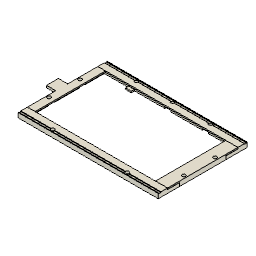
toshiba-screen-frame (Autodesk Fusion 360 design; units mm, degrees)
part number: 2026-06-13-12-57-34-662
part number: 2026-06-16-20-14-57-476
part number: 2026-06-16-20-14-57-486
part number: 2026-06-16-20-14-57-489
part number: 2026-06-16-20-14-57-492
part number: 2026-06-18-16-57-17-201
Autodesk Fusion 360 part; units mm, degrees
note: some values were not read from the file. Chosen so that the rebuilt part matches the saved one: which bodies a step acts on; which face or edge a step refers to. Set by a fixed rule: which sketch regions a step uses.
sketch "Main" plane through (0, 0, 0) normal (0, 1, 0) x (1, 0, 0)
  line L0 (0, 0) -> (200, 0)
  line L1 (200, 0) -> (200, -117)
  line L2 (200, -117) -> (0, -117)
  line L3 (0, -117) -> (0, 0)
  line L4 (-5, 3) -> (207, 3)
  line L5 (207, 3) -> (207, -124)
  line L6 (207, -124) -> (-5, -124)
  line L7 (-5, -124) -> (-5, 3)
  line L8 (-13, 15.5) -> (220.2, 15.5)
  line L9 (220.2, 15.5) -> (220.2, -132.5)
  line L10 (220.2, -132.5) -> (-13, -132.5)
  line L11 (-13, -132.5) -> (-13, 15.5)
  dimension "d1" = 200
  dimension "d2" = 117
  dimension "d4" = 127
  dimension "d5" = 3
  dimension "d6" = 5
  dimension "d7" = 148
  dimension "d9" = 12.5
  dimension "d10" = 8
  dimension "d37" = 7
  dimension "d38" = 212
  dimension "d39" = 13.2
  dimension "d40" = 233.2
  constraint horizontal L0
  constraint vertical L1
  constraint horizontal L2
  constraint vertical L3
  constraint coincident L0.start L3.end
  constraint horizontal L4
  constraint vertical L5
  constraint horizontal L6
  constraint vertical L7
  constraint horizontal L8
  constraint vertical L9
  constraint horizontal L10
  constraint vertical L11
  measures "d1" distance of L0.start L0.end
  measures "d2" distance of L0.start L2.end
  measures "d4" distance of L4.start L6.end
  measures "d5" distance of L0 L4
  measures "d6" distance of L3 L7
  measures "d7" distance of L8.start L10.end
  measures "d9" distance of L4 L8
  measures "d10" distance of L7 L11
  measures "d37" distance of L1 L5
  measures "d38" distance of L5 L7
  measures "d39" distance of L5 L9
  measures "d40" distance of L9 L11
extrude "Extrude1" add sketch "Main" against normal blind 7.9 contours L8 L9 L10 L11 makes body 1
extrude "Extrude2" add sketch "Main" against normal blind 2 contours L4 L5 L6 L7 bodies 1
sketch "Notches" plane through (0, -7.9, 0) normal (0, -1, 0) x (1, 0, 0)
  line L0 (-5, 124) -> (207, 124)
  line L1 (207, 124) -> (207, -3)
  line L2 (207, -3) -> (-5, -3)
  line L3 (-5, -3) -> (-5, 124)
  line L4 (220.2, 132.5) -> (-13, 132.5)
  line L5 (-13, 132.5) -> (-13, -15.5)
  line L6 (-13, -15.5) -> (220.2, -15.5)
  line L7 (220.2, -15.5) -> (220.2, 132.5)
  line L8 (35.1303, -3) -> (45.1303, -3)
  line L9 (45.1303, -3) -> (45.1303, -14)
  line L10 (45.1303, -14) -> (35.1303, -14)
  line L11 (35.1303, -14) -> (35.1303, -3)
  line L12 (95.4758, -3) -> (105.4758, -3)
  line L13 (105.4758, -3) -> (105.4758, -14)
  line L14 (105.4758, -14) -> (95.4758, -14)
  line L15 (95.4758, -14) -> (95.4758, -3)
  line L16 (158.4262, -3) -> (168.4262, -3)
  line L17 (168.4262, -3) -> (168.4262, -14)
  line L18 (168.4262, -14) -> (158.4262, -14)
  line L19 (158.4262, -14) -> (158.4262, -3)
  line L20 (-12, 90) -> (-5, 90)
  line L21 (-5, 90) -> (-5, 80)
  line L22 (-5, 80) -> (-12, 80)
  line L23 (-12, 80) -> (-12, 90)
  line L24 (-12, 38.3982) -> (-5, 38.3982)
  line L25 (-5, 38.3982) -> (-5, 28.3982)
  line L26 (-5, 28.3982) -> (-12, 28.3982)
  line L27 (-12, 28.3982) -> (-12, 38.3982)
  line L28 (34.9856, 124) -> (44.9856, 124)
  line L29 (44.9856, 124) -> (44.9856, 131)
  line L30 (44.9856, 131) -> (34.9856, 131)
  line L31 (34.9856, 131) -> (34.9856, 124)
  line L32 (158.8604, 124) -> (168.8604, 124)
  line L33 (168.8604, 124) -> (168.8604, 131)
  line L34 (168.8604, 131) -> (158.8604, 131)
  line L35 (158.8604, 131) -> (158.8604, 124)
  line L36 (207, 90.4116) -> (218.7, 90.4116)
  line L37 (218.7, 90.4116) -> (218.7, 80.4116)
  line L38 (218.7, 80.4116) -> (207, 80.4116)
  line L39 (207, 80.4116) -> (207, 90.4116)
  line L40 (207, 38.4594) -> (218.7, 38.4594)
  line L41 (218.7, 38.4594) -> (218.7, 28.4594)
  line L42 (218.7, 28.4594) -> (207, 28.4594)
  line L43 (207, 28.4594) -> (207, 38.4594)
  dimension "d15" = 10
  dimension "d17" = 10
  dimension "d19" = 10
  dimension "d21" = 10
  dimension "d22" = 10
  dimension "d23" = 10
  dimension "d27" = 10
  dimension "d29" = 10
  dimension "d30" = 10
  dimension "d62" = 1.5
  dimension "d63" = 1.5
  dimension "d64" = 1.5
  dimension "d65" = 1.5
  dimension "d66" = 1.5
  dimension "d67" = 1.5
  dimension "d68" = 1.5
  dimension "d71" = 7
  dimension "d72" = 7
  constraint horizontal L8
  constraint vertical L9
  constraint horizontal L10
  constraint vertical L11
  constraint horizontal L12
  constraint vertical L13
  constraint horizontal L14
  constraint vertical L15
  constraint horizontal L16
  constraint vertical L17
  constraint horizontal L18
  constraint vertical L19
  constraint horizontal L20
  constraint vertical L21
  constraint horizontal L22
  constraint vertical L23
  constraint horizontal L24
  constraint vertical L25
  constraint horizontal L26
  constraint vertical L27
  constraint horizontal L28
  constraint vertical L29
  constraint horizontal L30
  constraint vertical L31
  constraint horizontal L32
  constraint vertical L33
  constraint horizontal L34
  constraint vertical L35
  constraint horizontal L36
  constraint vertical L37
  constraint horizontal L38
  constraint vertical L39
  constraint horizontal L40
  constraint vertical L41
  constraint horizontal L42
  constraint vertical L43
  constraint collinear L2 L16
  constraint collinear L2 L8
  constraint collinear L2 L12
  constraint collinear L1 L43
  constraint collinear L1 L39
  constraint collinear L0 L32
  constraint collinear L0 L28
  constraint collinear L3 L25
  constraint collinear L3 L21
  measures "d15" distance of L8.start L8.end
  measures "d17" distance of L12.start L12.end
  measures "d19" distance of L16.start L16.end
  measures "d21" distance of L20.start L22.end
  measures "d22" distance of L24.start L26.end
  measures "d23" distance of L28.start L28.end
  measures "d27" distance of L32.start L32.end
  measures "d29" distance of L36.start L38.end
  measures "d30" distance of L40.start L42.end
  measures "d62" distance of L6 L18
  measures "d63" distance of L6 L14
  measures "d64" distance of L6 L10
  measures "d65" distance of L7 L41
  measures "d66" distance of L7 L37
  measures "d67" distance of L4 L34
  measures "d68" distance of L4 L30
  measures "d71" distance of L25 L27
  measures "d72" distance of L21 L23
extrude "Extrude3" cut sketch "Notches" against normal blind 2.3 contours L3 L20 L21 L22 L23 bodies 1
extrude "Extrude4" cut sketch "Notches" against normal blind 2.3 contours L0 L28 L29 L30 L31 | L0 L32 L33 L34 L35 | L3 L24 L25 L26 L27 | L1 L36 L37 L38 L39 | L2 L8 L9 L10 L11 | L1 L40 L41 L42 L43 | L2 L12 L13 L14 L15 | L2 L16 L17 L18 L19 bodies 1
ref_plane "WorkPlane1" through (103.6, -3.95, 102.5) normal (0, 0, 1) x (-1, 0, 0)
split "Split1" by plane through (103.6, -3.95, 102.5) normal (0, 0, 1) bodies 1 makes body 2 at (135.7333, 0, 127.3333)
ref_plane "WorkPlane2" through (103.6, -3.95, 14.5) normal (0, 0, -1) x (1, 0, 0)
split "Split2" by plane through (103.6, -3.95, 14.5) normal (0, 0, -1) bodies 1 makes body 3 at (206.7333, 0, 43.8333) makes body 4 at (135.7333, 0, -10.3333)
sketch "channels" plane through (220.2, 0, 0) normal (1, 0, 0) x (0, 0, -1)
  line L0 (-14.5, 0) -> (-14.5, -7.9)
  line L1 (-14.5, -7.9) -> (15.5, -7.9)
  line L2 (15.5, -7.9) -> (15.5, 0)
  line L3 (15.5, 0) -> (-14.5, 0)
  line L4 (14.5, 0) -> (11, 0)
  line L5 (11, 0) -> (11, -1)
  line L6 (11, -1) -> (14.5, -1)
  line L7 (14.5, -1) -> (14.5, 0)
  line L8 (-131.5, 0) -> (-128, 0)
  line L9 (-128, 0) -> (-128, -1)
  line L10 (-128, -1) -> (-131.5, -1)
  line L11 (-131.5, -1) -> (-131.5, 0)
  line L12 (-132.5, 0) -> (-132.5, -7.9)
  dimension "d41" = 3.5
  dimension "d42" = 1
  dimension "d43" = 1
  dimension "d44" = 3.5
  dimension "d45" = 1
  dimension "d46" = 1
  constraint horizontal L4
  constraint vertical L5
  constraint horizontal L6
  constraint vertical L7
  constraint coincident L3 L4.start
  constraint horizontal L8
  constraint vertical L9
  constraint horizontal L10
  constraint vertical L11
  measures "d41" distance of L4.start L4.end
  measures "d42" distance of L4.start L6.end
  measures "d43" distance of L2 L7
  measures "d44" distance of L8.start L8.end
  measures "d45" distance of L8.start L10.end
  measures "d46" distance of L11 L12
extrude "Extrude5" cut sketch "channels" against normal up to surface (233.2 mm away) contours L3 L4 L5 L6 L7 bodies 4
extrude "Extrude6" cut sketch "channels" against normal up to surface (233.2 mm away) contours L8 L9 L10 L11 bodies 2
combine "Combine1" operation add target body 4 tool bodies 3 2 1
ref_plane "WorkPlane5" through (163.4262, -4.1, -8.5) normal (0, -1, 0) x (0, 0, -1)
sketch "Screws Nuts" plane through (0, -4.1, 0) normal (0, -1, 0) x (-1, 0, 0)
  circle A0 centre (-163.4262, 11) radius 1.6
  circle A1 centre (-163.4262, 11) radius 2.85
  line L0 (-168.4262, 14) -> (-158.4262, 14)
  line L1 (-168.4262, 3) -> (-168.4262, 14)
  circle A2 centre (-100.4758, 11) radius 1.6
  circle A3 centre (-100.4758, 11) radius 2.85
  circle A4 centre (-40.1303, 11) radius 1.6
  circle A5 centre (-40.1303, 11) radius 2.85
  circle A6 centre (9, -33.3982) radius 1.6
  circle A7 centre (9, -33.3982) radius 2.85
  circle A8 centre (-215.7, -33.4594) radius 1.6
  circle A9 centre (-215.7, -33.4594) radius 2.85
  circle A10 centre (9, -85) radius 1.6
  circle A11 centre (9, -85) radius 2.85
  circle A12 centre (-215.7, -85.4116) radius 1.6
  circle A13 centre (-215.7, -85.4116) radius 2.85
  circle A14 centre (-163.8604, -128) radius 1.6
  circle A15 centre (-163.8604, -128) radius 2.85
  circle A16 centre (-39.9856, -128) radius 1.6
  circle A17 centre (-39.9856, -128) radius 2.85
  line L2 (-105.4758, 14) -> (-95.4758, 14)
  line L3 (-105.4758, 3) -> (-105.4758, 14)
  line L4 (-45.1303, 14) -> (-35.1303, 14)
  line L5 (-45.1303, 3) -> (-45.1303, 14)
  line L6 (12, -28.3982) -> (12, -38.3982)
  line L7 (5, -28.3982) -> (12, -28.3982)
  line L8 (12, -80) -> (12, -90)
  line L9 (5, -80) -> (12, -80)
  line L10 (-44.9856, -131) -> (-34.9856, -131)
  line L11 (-44.9856, -124) -> (-44.9856, -131)
  line L12 (-168.8604, -131) -> (-158.8604, -131)
  line L13 (-168.8604, -124) -> (-168.8604, -131)
  line L14 (-218.7, -90.4116) -> (-218.7, -80.4116)
  line L15 (-218.7, -80.4116) -> (-207, -80.4116)
  line L16 (-218.7, -38.4594) -> (-218.7, -28.4594)
  line L17 (-218.7, -28.4594) -> (-207, -28.4594)
  dimension "d74" = 3.2
  dimension "d75" = 5.7
  dimension "d76" = 3
  dimension "d77" = 5
  dimension "d82" = 3.2
  dimension "d83" = 5.7
  dimension "d84" = 3.2
  dimension "d85" = 5.7
  dimension "d86" = 3.2
  dimension "d87" = 5.7
  dimension "d88" = 3.2
  dimension "d89" = 5.7
  dimension "d90" = 3.2
  dimension "d91" = 5.7
  dimension "d92" = 3.2
  dimension "d93" = 5.7
  dimension "d94" = 3.2
  dimension "d95" = 5.7
  dimension "d96" = 3.2
  dimension "d97" = 5.7
  dimension "d98" = 3
  dimension "d99" = 5
  dimension "d100" = 3
  dimension "d101" = 5
  dimension "d102" = 3
  dimension "d103" = 5
  dimension "d104" = 3
  dimension "d105" = 5
  dimension "d106" = 3
  dimension "d107" = 5
  dimension "d108" = 3
  dimension "d109" = 5
  dimension "d110" = 3
  dimension "d111" = 5
  dimension "d112" = 3
  dimension "d113" = 5
  constraint concentric A0 A1
  constraint concentric A2 A3
  constraint concentric A4 A5
  constraint concentric A6 A7
  constraint concentric A8 A9
  constraint concentric A10 A11
  constraint concentric A12 A13
  constraint concentric A14 A15
  constraint concentric A16 A17
  measures "d74" diameter of A0
  measures "d75" diameter of A1
  measures "d76" distance of A0.centre L0
  measures "d77" distance of A0.centre L1
  measures "d82" diameter of A2
  measures "d83" diameter of A3
  measures "d84" diameter of A4
  measures "d85" diameter of A5
  measures "d86" diameter of A6
  measures "d87" diameter of A7
  measures "d88" diameter of A8
  measures "d89" diameter of A9
  measures "d90" diameter of A10
  measures "d91" diameter of A11
  measures "d92" diameter of A12
  measures "d93" diameter of A13
  measures "d94" diameter of A14
  measures "d95" diameter of A15
  measures "d96" diameter of A16
  measures "d97" diameter of A17
  measures "d98" distance of A2.centre L2
  measures "d99" distance of A2.centre L3
  measures "d100" distance of A4.centre L4
  measures "d101" distance of A4.centre L5
  measures "d102" distance of A6.centre L6
  measures "d103" distance of A6.centre L7
  measures "d104" distance of A10.centre L8
  measures "d105" distance of A10.centre L9
  measures "d106" distance of A16.centre L10
  measures "d107" distance of A16.centre L11
  measures "d108" distance of A14.centre L12
  measures "d109" distance of A14.centre L13
  measures "d110" distance of A12.centre L14
  measures "d111" distance of A12.centre L15
  measures "d112" distance of A8.centre L16
  measures "d113" distance of A8.centre L17
extrude "Extrude11" cut sketch "Screws Nuts" along normal up to surface (3.8 mm away) contours A0 | A2 | A4 | A6 | A8 | A10 | A12 | A14 | A16 bodies 4
extrude "Extrude12" cut sketch "Screws Nuts" against normal up to surface (4.1 mm away) contours A0 | A1 | A2 | A3 | A4 | A5 | A6 | A7 | A8 | A9 | A10 | A11 | A12 | A13 | A14 | A15 | A16 | A17 bodies 4
sketch "body cuts" plane through (-13, 0, 0) normal (-1, 0, 0) x (0, 0, 1)
  line L0 (-14.5, -1) -> (-14.5, 0)
  line L1 (-14.5, 0) -> (-15.5, 0)
  line L2 (-15.5, 0) -> (-15.5, -7.9)
  line L3 (-15.5, -7.9) -> (132.5, -7.9)
  line L4 (132.5, -7.9) -> (132.5, 0)
  line L5 (132.5, 0) -> (131.5, 0)
  line L6 (131.5, 0) -> (131.5, -1)
  line L7 (131.5, -1) -> (128, -1)
  line L8 (128, -1) -> (128, 0)
  line L9 (128, 0) -> (-11, 0)
  line L10 (-11, 0) -> (-11, -1)
  line L11 (-11, -1) -> (-14.5, -1)
  line L12 (0, 0) -> (0, -2)
  line L13 (0, -2) -> (20, -2)
  line L14 (20, -2) -> (20, -7.9)
  line L15 (117, 0) -> (117, -2)
  line L16 (117, -2) -> (97, -2)
  line L17 (97, -2) -> (97, -7.9)
  constraint coincident L12.start origin
  constraint perpendicular L9 L12
  constraint perpendicular L12 L13
  constraint coincident L3 L14.end
  constraint perpendicular L3 L14
  constraint coincident L9 L15.start
  constraint perpendicular L9 L15
  constraint perpendicular L15 L16
  constraint coincident L3 L17.end
  constraint perpendicular L3 L17
split "Split5" by curves path "body cuts" along L15 L16 L17 L12 L13 L14 bodies 4 makes body 5 at (211.7553, 0, 10.227) makes body 6 at (-7.2623, 0, 10.1854) makes body 7 at (215.8, -7.9, 0.5)
sketch "Registr Pegs" plane through (0, -2, 0) normal (0, -1, 0) x (1, 0, 0)
  line L0 (-5, 117) -> (207, 117)
  line L1 (207, 117) -> (207, 124)
  line L2 (207, 124) -> (-5, 124)
  line L3 (-5, 124) -> (-5, 117)
  circle A0 centre (-9, 15) radius 1.75
  circle A1 centre (-9, 4) radius 1.75
  circle A2 centre (-9, 15) radius 2
  circle A3 centre (-9, 4) radius 2
  circle A4 centre (-9, 101) radius 2
  circle A5 centre (-9, 101) radius 1.75
  circle A6 centre (-9, 112) radius 2
  circle A7 centre (-9, 112) radius 1.75
  circle A8 centre (214, 101) radius 2
  circle A9 centre (214, 101) radius 1.75
  circle A10 centre (214, 112) radius 2
  circle A11 centre (214, 112) radius 1.75
  circle A12 centre (214, 4) radius 2
  circle A13 centre (214, 4) radius 1.75
  circle A14 centre (214, 15.5) radius 2
  circle A15 centre (214, 15.5) radius 1.75
  dimension "d118" = 3.5
  dimension "d119" = 3.5
  dimension "d120" = 4
  dimension "d121" = 4
  dimension "d130" = 3.5
  dimension "d131" = 4
  dimension "d132" = 3.5
  dimension "d133" = 4
  dimension "d134" = 3.5
  dimension "d135" = 4
  dimension "d136" = 3.5
  dimension "d137" = 4
  dimension "d138" = 3.5
  dimension "d139" = 4
  dimension "d140" = 3.5
  dimension "d141" = 4
  constraint concentric A0 A2
  constraint concentric A1 A3
  constraint concentric A4 A5
  constraint concentric A6 A7
  constraint concentric A8 A9
  constraint concentric A10 A11
  constraint concentric A12 A13
  constraint concentric A14 A15
  measures "d118" diameter of A0
  measures "d119" diameter of A1
  measures "d120" diameter of A2
  measures "d121" diameter of A3
  measures "d130" diameter of A5
  measures "d131" diameter of A4
  measures "d132" diameter of A7
  measures "d133" diameter of A6
  measures "d134" diameter of A9
  measures "d135" diameter of A8
  measures "d136" diameter of A11
  measures "d137" diameter of A10
  measures "d138" diameter of A13
  measures "d139" diameter of A12
  measures "d140" diameter of A15
  measures "d141" diameter of A14
extrude "top peg holes" cut sketch "Registr Pegs" along normal up to surface (5.9 mm away) contours A0 | A1 | A2 | A3 | A12 | A13 | A14 | A15 bodies 7
extrude "bot peg holes" cut sketch "Registr Pegs" along normal up to surface (5.9 mm away) contours A4 | A5 | A6 | A7 | A8 | A9 | A10 | A11 bodies 4
extrude "pegs" add sketch "Registr Pegs" along normal blind 8 contours A0 | A1 | A5 | A7 | A9 | A11 | A13 | A15 bodies 5 6
ref_plane "WorkPlane6" through (12, -3.95, 58.5) normal (-1, 0, 0) x (0, 0, -1)
ref_plane "WorkPlane7" through (103.6, -3.95, 24.5) normal (0, 0, -1) x (1, 0, 0)
extrude "width correction" cut 4 faces at (208.7327, -2, 108.3774) (-8.9502, -2, 115.9981) (208.7327, -2, 11.5441) (-8.9502, -2, 18.9981) along direction (0, -1, 0) blind 0.2 on bodies 4 7 bodies 4 7
copy_body "Body->Comp1" bodies 4 removing the originals makes body 8 in component "Bottom"
copy_body "Body->Comp2" bodies 5 removing the originals makes body 9 in component "Right"
copy_body "Body->Comp3" bodies 6 removing the originals makes body 10 in component "Left"
copy_body "Body->Comp4" bodies 7 removing the originals makes body 11 in component "Top"
sketch "right stopper" plane through (-13, 0, 0) normal (-1, 0, 0) x (0, 0, 1)
  line L0 (20, -2) -> (20, -7.9)
  line L1 (20, -7.9) -> (97, -7.9)
  line L2 (97, -7.9) -> (97, -2)
  line L3 (97, -2) -> (117, -2)
  line L4 (117, -2) -> (117, 0)
  line L5 (117, 0) -> (0, 0)
  line L6 (0, 0) -> (0, -2)
  line L7 (0, -2) -> (20, -2)
  line L8 (69.8728, -3.7674) -> (49.8728, -3.7674)
  line L9 (49.8728, -3.7674) -> (49.8728, 0)
  line L10 (49.8728, 0) -> (69.8728, 0)
  line L11 (69.8728, 0) -> (69.8728, -3.7674)
  dimension "d146" = 20
  constraint horizontal L8
  constraint vertical L9
  constraint horizontal L10
  constraint vertical L11
  measures "d146" distance of L8.start L8.end
extrude "right stopper" add sketch "right stopper" along normal blind 15.5 contours L5 L8 L9 L10 L11 bodies 10 in component "Left"
fillet "Fillet1" [suppressed] in component "Left"
sketch "clamp" plane through (0, -5.6, 0) normal (0, -1, 0) x (1, 0, 0)
  circle A0 centre (215.7, 33.4594) radius 1.6
  line L0 (207, 28.4594) -> (218.7, 28.4594)
  line L1 (218.7, 28.4594) -> (218.7, 38.4594)
  line L2 (218.7, 38.4594) -> (207, 38.4594)
  line L3 (207, 38.4594) -> (207, 28.4594)
  line L4 (45.1303, -14) -> (35.1303, -14)
  line L5 (35.1303, -14) -> (35.1303, 2.5)
  line L6 (35.1303, 2.5) -> (45.1303, 2.5)
  line L7 (45.1303, 2.5) -> (45.1303, -14)
  line L8 (45.1303, -3) -> (45.1303, -14)
  line L9 (35.1303, -14) -> (35.1303, -3)
  line L10 (45.1303, -14) -> (35.1303, -14)
  line L11 (35.2803, 2.35) -> (44.9803, 2.35)
  line L12 (44.9803, 2.35) -> (44.9803, -13.85)
  line L13 (44.9803, -13.85) -> (35.2803, -13.85)
  line L14 (35.2803, -13.85) -> (35.2803, 2.35)
  circle A1 centre (40.1303, -11) radius 1.6
  circle A2 centre (40.1303, -11) radius 1.6
  dimension "d157" = 16.5
  dimension "d158" = 0.15
  constraint horizontal L4
  constraint vertical L5
  constraint horizontal L6
  constraint vertical L7
  constraint collinear L7 L8
  constraint collinear L5 L9
  constraint collinear L4 L10
  constraint concentric A1 A2
  constraint equal A1 A2
  measures "d157" distance of L4.start L6.end
extrude "clamp body" add sketch "clamp" along normal up to surface (2.3 mm away) separate body contours L11 L12 L13 L14 | A1 A2 makes body 12
extrude "clamp hole" cut sketch "clamp" along normal through all contours A1 A2 bodies 12
copy_body "Body->Comp5" bodies 12 removing the originals makes body 13 in component "clamp"
sketch "clamp-notch" plane through (44.9803, 0, 0) normal (1, 0, 0) x (0, 0, -1)
  line L0 (-2.35, -7.9) -> (13.85, -7.9)
  line L1 (13.85, -7.9) -> (13.85, -5.6)
  line L2 (13.85, -5.6) -> (-2.35, -5.6)
  line L3 (-2.35, -5.6) -> (-2.35, -7.9)
  line L4 (1.6779, -7.9) -> (0.4779, -7.9)
  line L5 (0.4779, -7.9) -> (0.4779, -8.1)
  line L6 (0.4779, -8.1) -> (1.6779, -8.1)
  line L7 (1.6779, -8.1) -> (1.6779, -7.9)
  dimension "d162" = 1.2
  dimension "d163" = 0.2
  constraint horizontal L4
  constraint vertical L5
  constraint horizontal L6
  constraint vertical L7
  constraint coincident L0 L4.start
  measures "d162" distance of L4.start L4.end
  measures "d163" distance of L4.start L6.end
extrude "Extrude1'" add sketch "clamp-notch" against normal up to surface (9.7 mm away) contours L0 L4 L5 L6 L7 bodies 13 in component "clamp"
component "Bottom" placed x (1, 0, 0) y (0, 1, 0) z (0, 0, 1) at (0, 0, 0)
component "Right" placed x (1, 0, 0) y (0, 1, 0) z (0, 0, 1) at (0, 0, 0)
component "Left" placed x (1, 0, 0) y (0, 1, 0) z (0, 0, 1) at (0, 0, 0)
component "Top" placed x (1, 0, 0) y (0, 1, 0) z (0, 0, 1) at (0, 0, 0)
component "clamp" placed x (1, 0, 0) y (0, 1, 0) z (0, 0, 1) at (0, 0, 0)
equation "d4 = 3 mm + 117 mm + 7 mm"
equation "d7 = 12.5 mm + 127 mm + 8.5 mm"
equation "d39 = 14 mm - 0.8 mm"
named bodies: "Left", "Bottom", "Right", "Top"
